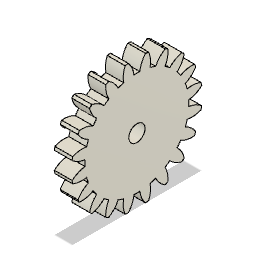
4 cm gear v5 (Autodesk Fusion 360 design; units mm, degrees)
Autodesk Fusion 360 part; units mm, degrees
sketch "Sketch1" plane through (0, 0, 0) normal (1, 0, 0) x (0, 0, -1)
  arc A0 (30.8871, 27.0565) -> (30.1313, 27.8123) centre (14.9574, 11.8827) ccw
  arc A1 (10.989, -9.7564) -> (12.0447, -9.9237) centre (14.9574, 11.8827) ccw
  arc A2 (4.4964, -7.4711) -> (5.4488, -7.9563) centre (14.9574, 11.8827) ccw
  arc A3 (12.0447, 33.689) -> (10.989, 33.5218) centre (14.9574, 11.8827) ccw
  arc A4 (24.4289, 26.5968) -> (25.4184, 31.2364) centre (17.4515, 30.5103) ccw
  arc A5 (34.3112, 22.3437) -> (29.6716, 21.3542) centre (33.5851, 14.3767) ccw
  arc A6 (25.4184, -7.4711) -> (24.4289, -2.8315) centre (17.4515, -6.745) ccw
  arc A7 (32.4286, 10.8965) -> (32.4286, 12.8689) centre (14.9574, 11.8827) ccw
  arc A8 (36.5965, 7.9143) -> (36.7638, 8.97) centre (14.9574, 11.8827) ccw
  arc A9 (30.8871, -3.2912) -> (28.5123, 0.8155) centre (23.0856, -5.0625) ccw
  arc A10 (1.4026, 0.8155) -> (-0.9722, -3.2912) centre (6.8292, -5.0625) ccw
  arc A11 (-1.3539, 18.2195) -> (-1.9634, 16.3437) centre (14.9574, 11.8827) ccw
  arc A12 (-2.5138, 12.8689) -> (-2.5138, 10.8965) centre (14.9574, 11.8827) ccw
  arc A13 (-1.9634, 16.3437) -> (-6.6817, 15.8511) centre (-3.5292, 8.4984) ccw
  arc A14 (28.5123, 0.8155) -> (29.6716, 2.4112) centre (14.9574, 11.8827) ccw
  arc A15 (10.989, -9.7564) -> (12.0447, -9.9237) centre (14.9574, 11.8827) ccw
  arc A16 (29.6716, 2.4112) -> (34.3112, 1.4217) centre (33.5851, 9.3886) ccw
  arc A17 (8.6206, -4.4287) -> (10.4964, -5.0382) centre (14.9574, 11.8827) ccw
  arc A18 (36.7638, 8.97) -> (32.4286, 10.8965) centre (31.4935, 2.9514) ccw
  arc A19 (28.5123, 0.8155) -> (29.6716, 2.4112) centre (14.9574, 11.8827) ccw
  arc A20 (5.4859, -2.8315) -> (4.4964, -7.4711) centre (12.4634, -6.745) ccw
  arc A21 (24.4661, 31.7217) -> (21.2942, 28.194) centre (28.5615, 24.8494) ccw
  arc A22 (-0.9722, 27.0565) -> (1.4026, 22.9498) centre (6.8292, 28.8279) ccw
  arc A23 (21.2942, -4.4287) -> (24.4661, -7.9563) centre (28.5615, -1.0841) ccw
  arc A24 (25.4184, 31.2364) -> (24.4661, 31.7217) centre (14.9574, 11.8827) ccw
  arc A25 (-1.3539, 5.5459) -> (-4.8816, 2.374) centre (1.9907, -1.7214) ccw
  arc A26 (25.4184, -7.4711) -> (24.4289, -2.8315) centre (17.4515, -6.745) ccw
  arc A27 (5.4859, 26.5968) -> (3.8903, 25.4375) centre (14.9574, 11.8827) ccw
  arc A28 (-0.9722, -3.2912) -> (-0.2164, -4.047) centre (14.9574, 11.8827) ccw
  arc A29 (-6.8489, 8.97) -> (-6.6817, 7.9143) centre (14.9574, 11.8827) ccw
  arc A30 (24.4661, -7.9563) -> (25.4184, -7.4711) centre (14.9574, 11.8827) ccw
  arc A31 (10.989, 33.5218) -> (10.4964, 28.8035) centre (18.3417, 30.3693) ccw
  arc A32 (-0.2164, -4.047) -> (3.8903, -1.6722) centre (-1.9878, 3.7545) ccw
  arc A33 (18.9258, 33.5218) -> (17.8701, 33.689) centre (14.9574, 11.8827) ccw
  arc A34 (3.8903, 25.4375) -> (-0.2164, 27.8123) centre (-1.9878, 20.0109) ccw
  arc A35 (12.0447, 33.689) -> (10.989, 33.5218) centre (14.9574, 11.8827) ccw
  arc A36 (0.2433, 2.4112) -> (1.4026, 0.8155) centre (14.9574, 11.8827) ccw
  arc A37 (-0.9722, 27.0565) -> (1.4026, 22.9498) centre (6.8292, 28.8279) ccw
  arc A38 (24.4289, -2.8315) -> (26.0246, -1.6722) centre (14.9574, 11.8827) ccw
  arc A39 (-6.8489, 8.97) -> (-6.6817, 7.9143) centre (14.9574, 11.8827) ccw
  arc A40 (-4.3963, 1.4217) -> (0.2433, 2.4112) centre (-3.6702, 9.3886) ccw
  arc A41 (1.4026, 0.8155) -> (-0.9722, -3.2912) centre (6.8292, -5.0625) ccw
  arc A42 (-0.2164, 27.8123) -> (-0.9722, 27.0565) centre (14.9574, 11.8827) ccw
  arc A43 (8.6206, 28.194) -> (5.4488, 31.7217) centre (1.3533, 24.8494) ccw
  arc A44 (4.4964, 31.2364) -> (5.4859, 26.5968) centre (12.4634, 30.5103) ccw
  arc A45 (0.2433, 21.3542) -> (-4.3963, 22.3437) centre (-3.6702, 14.3767) ccw
  arc A46 (18.9258, 33.5218) -> (17.8701, 33.689) centre (14.9574, 11.8827) ccw
  arc A47 (4.4964, 31.2364) -> (5.4859, 26.5968) centre (12.4634, 30.5103) ccw
  arc A48 (19.4184, 28.8035) -> (18.9258, 33.5218) centre (11.5731, 30.3693) ccw
  arc A49 (-1.9634, 7.4217) -> (-1.3539, 5.5459) centre (14.9574, 11.8827) ccw
  arc A50 (10.4964, -5.0382) -> (10.989, -9.7564) centre (18.3417, -6.604) ccw
  arc A51 (30.8871, 27.0565) -> (30.1313, 27.8123) centre (14.9574, 11.8827) ccw
  arc A52 (-4.8816, 2.374) -> (-4.3963, 1.4217) centre (14.9574, 11.8827) ccw
  arc A53 (21.2942, 28.194) -> (19.4184, 28.8035) centre (14.9574, 11.8827) ccw
  arc A54 (-0.9722, -3.2912) -> (-0.2164, -4.047) centre (14.9574, 11.8827) ccw
  arc A55 (30.1313, 27.8123) -> (26.0246, 25.4375) centre (31.9027, 20.0109) ccw
  arc A56 (-4.3963, 22.3437) -> (-4.8816, 21.3913) centre (14.9574, 11.8827) ccw
  arc A57 (13.9712, 29.3539) -> (12.0447, 33.689) centre (6.0261, 28.4187) ccw
  arc A58 (-2.5138, 10.8965) -> (-6.8489, 8.97) centre (-1.5786, 2.9514) ccw
  arc A59 (13.9712, 29.3539) -> (12.0447, 33.689) centre (6.0261, 28.4187) ccw
  arc A60 (34.7964, 21.3913) -> (34.3112, 22.3437) centre (14.9574, 11.8827) ccw
  arc A61 (8.6206, 28.194) -> (5.4488, 31.7217) centre (1.3533, 24.8494) ccw
  arc A62 (-2.5138, 12.8689) -> (-2.5138, 10.8965) centre (14.9574, 11.8827) ccw
  arc A63 (19.4184, -5.0382) -> (21.2942, -4.4287) centre (14.9574, 11.8827) ccw
  arc A64 (13.9712, -5.5885) -> (15.9436, -5.5885) centre (14.9574, 11.8827) ccw
  arc A65 (30.1313, 27.8123) -> (26.0246, 25.4375) centre (31.9027, 20.0109) ccw
  arc A66 (19.4184, 28.8035) -> (18.9258, 33.5218) centre (11.5731, 30.3693) ccw
  arc A67 (18.9258, -9.7564) -> (19.4184, -5.0382) centre (11.5731, -6.604) ccw
  arc A68 (-6.6817, 7.9143) -> (-1.9634, 7.4217) centre (-3.5292, 15.267) ccw
  arc A69 (5.4488, 31.7217) -> (4.4964, 31.2364) centre (14.9574, 11.8827) ccw
  arc A70 (12.0447, -9.9237) -> (13.9712, -5.5885) centre (6.0261, -4.6534) ccw
  arc A71 (36.7638, 14.7954) -> (36.5965, 15.8511) centre (14.9574, 11.8827) ccw
  arc A72 (32.4286, 12.8689) -> (36.7638, 14.7954) centre (31.4935, 20.814) ccw
  arc A73 (10.4964, 28.8035) -> (8.6206, 28.194) centre (14.9574, 11.8827) ccw
  arc A74 (15.9436, -5.5885) -> (17.8701, -9.9237) centre (23.8887, -4.6534) ccw
  arc A75 (17.8701, -9.9237) -> (18.9258, -9.7564) centre (14.9574, 11.8827) ccw
  arc A76 (1.4026, 22.9498) -> (0.2433, 21.3542) centre (14.9574, 11.8827) ccw
  arc A77 (26.0246, 25.4375) -> (24.4289, 26.5968) centre (14.9574, 11.8827) ccw
  arc A78 (17.8701, 33.689) -> (15.9436, 29.3539) centre (23.8887, 28.4187) ccw
  arc A79 (32.4286, 10.8965) -> (32.4286, 12.8689) centre (14.9574, 11.8827) ccw
  arc A80 (15.9436, 29.3539) -> (13.9712, 29.3539) centre (14.9574, 11.8827) ccw
  arc A81 (24.4289, 26.5968) -> (25.4184, 31.2364) centre (17.4515, 30.5103) ccw
  arc A82 (32.4286, 12.8689) -> (36.7638, 14.7954) centre (31.4935, 20.814) ccw
  arc A83 (25.4184, 31.2364) -> (24.4661, 31.7217) centre (14.9574, 11.8827) ccw
  arc A84 (36.7638, 14.7954) -> (36.5965, 15.8511) centre (14.9574, 11.8827) ccw
  arc A85 (34.7964, 21.3913) -> (34.3112, 22.3437) centre (14.9574, 11.8827) ccw
  arc A86 (31.2688, 18.2195) -> (34.7964, 21.3913) centre (27.9242, 25.4868) ccw
  arc A87 (28.5123, 22.9498) -> (30.8871, 27.0565) centre (23.0856, 28.8279) ccw
  arc A88 (34.3112, 22.3437) -> (29.6716, 21.3542) centre (33.5851, 14.3767) ccw
  arc A89 (31.8783, 16.3437) -> (31.2688, 18.2195) centre (14.9574, 11.8827) ccw
  arc A90 (36.5965, 15.8511) -> (31.8783, 16.3437) centre (33.4441, 8.4984) ccw
  arc A91 (29.6716, 21.3542) -> (28.5123, 22.9498) centre (14.9574, 11.8827) ccw
  arc A92 (-4.8816, 21.3913) -> (-1.3539, 18.2195) centre (1.9907, 25.4868) ccw
  arc A93 (4.4964, -7.4711) -> (5.4488, -7.9563) centre (14.9574, 11.8827) ccw
  arc A94 (30.1313, -4.047) -> (30.8871, -3.2912) centre (14.9574, 11.8827) ccw
  arc A95 (5.4859, -2.8315) -> (4.4964, -7.4711) centre (12.4634, -6.745) ccw
  arc A96 (5.4488, -7.9563) -> (8.6206, -4.4287) centre (1.3533, -1.0841) ccw
  arc A97 (26.0246, -1.6722) -> (30.1313, -4.047) centre (31.9027, 3.7545) ccw
  arc A98 (-1.3539, 18.2195) -> (-1.9634, 16.3437) centre (14.9574, 11.8827) ccw
  arc A99 (10.989, 33.5218) -> (10.4964, 28.8035) centre (18.3417, 30.3693) ccw
  arc A100 (30.1313, -4.047) -> (30.8871, -3.2912) centre (14.9574, 11.8827) ccw
  arc A101 (-4.3963, 22.3437) -> (-4.8816, 21.3913) centre (14.9574, 11.8827) ccw
  arc A102 (21.2942, -4.4287) -> (24.4661, -7.9563) centre (28.5615, -1.0841) ccw
  arc A103 (15.9436, -5.5885) -> (17.8701, -9.9237) centre (23.8887, -4.6534) ccw
  arc A104 (29.6716, 2.4112) -> (34.3112, 1.4217) centre (33.5851, 9.3886) ccw
  arc A105 (18.9258, -9.7564) -> (19.4184, -5.0382) centre (11.5731, -6.604) ccw
  arc A106 (3.8903, -1.6722) -> (5.4859, -2.8315) centre (14.9574, 11.8827) ccw
  arc A107 (31.8783, 7.4217) -> (36.5965, 7.9143) centre (33.4441, 15.267) ccw
  arc A108 (34.3112, 1.4217) -> (34.7964, 2.374) centre (14.9574, 11.8827) ccw
  arc A109 (1.4026, 22.9498) -> (0.2433, 21.3542) centre (14.9574, 11.8827) ccw
  arc A110 (0.2433, 21.3542) -> (-4.3963, 22.3437) centre (-3.6702, 14.3767) ccw
  arc A111 (34.7964, 2.374) -> (31.2688, 5.5459) centre (27.9242, -1.7214) ccw
  arc A112 (24.4661, -7.9563) -> (25.4184, -7.4711) centre (14.9574, 11.8827) ccw
  arc A113 (26.0246, -1.6722) -> (30.1313, -4.047) centre (31.9027, 3.7545) ccw
  arc A114 (31.2688, 5.5459) -> (31.8783, 7.4217) centre (14.9574, 11.8827) ccw
  arc A115 (10.4964, -5.0382) -> (10.989, -9.7564) centre (18.3417, -6.604) ccw
  arc A116 (12.0447, -9.9237) -> (13.9712, -5.5885) centre (6.0261, -4.6534) ccw
  arc A117 (-6.6817, 15.8511) -> (-6.8489, 14.7954) centre (14.9574, 11.8827) ccw
  arc A118 (34.3112, 1.4217) -> (34.7964, 2.374) centre (14.9574, 11.8827) ccw
  arc A119 (24.4289, -2.8315) -> (26.0246, -1.6722) centre (14.9574, 11.8827) ccw
  arc A120 (-6.8489, 14.7954) -> (-2.5138, 12.8689) centre (-1.5786, 20.814) ccw
  arc A121 (-4.8816, 2.374) -> (-4.3963, 1.4217) centre (14.9574, 11.8827) ccw
  arc A122 (10.4964, 28.8035) -> (8.6206, 28.194) centre (14.9574, 11.8827) ccw
  arc A123 (5.4859, 26.5968) -> (3.8903, 25.4375) centre (14.9574, 11.8827) ccw
  arc A124 (36.5965, 7.9143) -> (36.7638, 8.97) centre (14.9574, 11.8827) ccw
  arc A125 (3.8903, -1.6722) -> (5.4859, -2.8315) centre (14.9574, 11.8827) ccw
  arc A126 (-2.5138, 10.8965) -> (-6.8489, 8.97) centre (-1.5786, 2.9514) ccw
  arc A127 (5.4488, 31.7217) -> (4.4964, 31.2364) centre (14.9574, 11.8827) ccw
  arc A128 (-4.3963, 1.4217) -> (0.2433, 2.4112) centre (-3.6702, 9.3886) ccw
  arc A129 (34.7964, 2.374) -> (31.2688, 5.5459) centre (27.9242, -1.7214) ccw
  arc A130 (13.9712, -5.5885) -> (15.9436, -5.5885) centre (14.9574, 11.8827) ccw
  arc A131 (-6.6817, 7.9143) -> (-1.9634, 7.4217) centre (-3.5292, 15.267) ccw
  arc A132 (31.8783, 7.4217) -> (36.5965, 7.9143) centre (33.4441, 15.267) ccw
  arc A133 (5.4488, -7.9563) -> (8.6206, -4.4287) centre (1.3533, -1.0841) ccw
  arc A134 (0.2433, 2.4112) -> (1.4026, 0.8155) centre (14.9574, 11.8827) ccw
  arc A135 (36.7638, 8.97) -> (32.4286, 10.8965) centre (31.4935, 2.9514) ccw
  arc A136 (-0.2164, -4.047) -> (3.8903, -1.6722) centre (-1.9878, 3.7545) ccw
  arc A137 (28.5123, 22.9498) -> (30.8871, 27.0565) centre (23.0856, 28.8279) ccw
  arc A138 (19.4184, -5.0382) -> (21.2942, -4.4287) centre (14.9574, 11.8827) ccw
  arc A139 (17.8701, -9.9237) -> (18.9258, -9.7564) centre (14.9574, 11.8827) ccw
  arc A140 (30.8871, -3.2912) -> (28.5123, 0.8155) centre (23.0856, -5.0625) ccw
  arc A141 (21.2942, 28.194) -> (19.4184, 28.8035) centre (14.9574, 11.8827) ccw
  arc A142 (36.5965, 15.8511) -> (31.8783, 16.3437) centre (33.4441, 8.4984) ccw
  arc A143 (-1.9634, 16.3437) -> (-6.6817, 15.8511) centre (-3.5292, 8.4984) ccw
  arc A144 (-6.8489, 14.7954) -> (-2.5138, 12.8689) centre (-1.5786, 20.814) ccw
  arc A145 (29.6716, 21.3542) -> (28.5123, 22.9498) centre (14.9574, 11.8827) ccw
  arc A146 (8.6206, -4.4287) -> (10.4964, -5.0382) centre (14.9574, 11.8827) ccw
  arc A147 (-4.8816, 21.3913) -> (-1.3539, 18.2195) centre (1.9907, 25.4868) ccw
  arc A148 (26.0246, 25.4375) -> (24.4289, 26.5968) centre (14.9574, 11.8827) ccw
  arc A149 (3.8903, 25.4375) -> (-0.2164, 27.8123) centre (-1.9878, 20.0109) ccw
  arc A150 (17.8701, 33.689) -> (15.9436, 29.3539) centre (23.8887, 28.4187) ccw
  arc A151 (-1.9634, 7.4217) -> (-1.3539, 5.5459) centre (14.9574, 11.8827) ccw
  arc A152 (15.9436, 29.3539) -> (13.9712, 29.3539) centre (14.9574, 11.8827) ccw
  arc A153 (31.8783, 16.3437) -> (31.2688, 18.2195) centre (14.9574, 11.8827) ccw
  arc A154 (-6.6817, 15.8511) -> (-6.8489, 14.7954) centre (14.9574, 11.8827) ccw
  arc A155 (-1.3539, 5.5459) -> (-4.8816, 2.374) centre (1.9907, -1.7214) ccw
  arc A156 (24.4661, 31.7217) -> (21.2942, 28.194) centre (28.5615, 24.8494) ccw
  arc A157 (-0.2164, 27.8123) -> (-0.9722, 27.0565) centre (14.9574, 11.8827) ccw
  arc A158 (31.2688, 18.2195) -> (34.7964, 21.3913) centre (27.9242, 25.4868) ccw
  arc A159 (31.2688, 5.5459) -> (31.8783, 7.4217) centre (14.9574, 11.8827) ccw
  circle A160 centre (14.9574, 11.8827) radius 2.75
  dimension "d4" = 5.5
  constraint concentric A145 A160
  measures "d4" diameter of A160
extrude "Extrude1" add sketch "Sketch1" along normal blind 6
